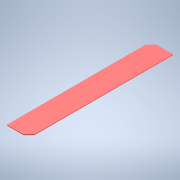
# Autodesk Inventor part: VPTrack
Saved by Autodesk Inventor 2021 (Build 250183000, 183)
## iProperties
Created: 2023-03-16
Part Number: VPTrack
Material: Paper
Document SubType Name: Modeling
Designer: Bradley
Density: 0.93 g/cm^3
Appearance: Smooth - Red
Author: Bradley
Autodesk Inventor part; units mm, degrees
ref_plane "YZ Plane" through (0, 0, 0) normal (1, 0, 0) x (0, 1, 0)
ref_plane "XZ Plane" through (0, 0, 0) normal (0, 1, 0) x (-1, 0, 0)
ref_plane "XY Plane" through (0, 0, 0) normal (0, 0, 1) x (1, 0, 0)
sketch "Sketch1" plane through (0, 0, 0) normal (0, 1, 0) x (-1, 0, 0)
  line L0 (-19, 125.5) -> (19, 125.5)
  line L1 (19, 125.5) -> (19, -125.5)
  line L2 (19, -125.5) -> (-19, -125.5)
  line L3 (-19, -125.5) -> (-19, 125.5)
  line L4 (-19, 125.5) -> (19, -125.5) construction
  line L5 (19, 125.5) -> (-19, -125.5) construction
  line L6 (-9, 125.5) -> (-19, 115.5)
  line L7 (9, -125.5) -> (19, -115.5)
  point P0 (0, 0)
  dimension "d0" = 38
  dimension "d1" = 251
  dimension "d2" = 10
  dimension "d3" = 10
  constraints: 16 end point, 4 parallel, 4 point on line, 2 midpoint, 1 horizontal, 1 perpendicular
  measures "d0" distance of L1.end L2.end
  measures "d1" distance of L0.end L1.end
  measures "d2" horizontal distance of L7.start L7.end
  measures "d3" horizontal distance of L7.start L7.end
extrude "Extrusion1" add sketch "Sketch1" along normal mid plane 1.7 contours L0 L1 L7 L2 L3 L6
equation "\"d3\" = d2"
body "Solid1"
